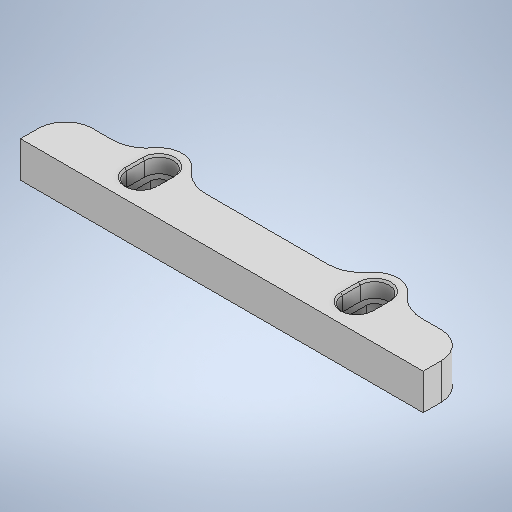
# Autodesk Inventor part: Montagemodul
Saved by Autodesk Inventor 2025.2 (Build 292293000, 293)
## iProperties
Created: 2025-11-06
Part Number: Montagemodul
Material: Generisch
Document SubType Name: Modeling
Designer: leowa
Density: 1 g/cm^3
Appearance: Vorgabe
Author: leowa
Autodesk Inventor part; units mm, degrees
ref_plane "YZ Plane" through (0, 0, 0) normal (1, 0, 0) x (0, 1, 0)
ref_plane "XZ Plane" through (0, 0, 0) normal (0, 1, 0) x (-1, 0, 0)
ref_plane "XY Plane" through (0, 0, 0) normal (0, 0, 1) x (1, 0, 0)
sketch "Skizze1" plane through (0, 0, 0) normal (0, 1, 0) x (-1, 0, 0)
  line L0 (-56, 7.5) -> (56, 7.5)
  line L1 (56, 7.5) -> (56, -7.5)
  line L2 (56, -7.5) -> (-56, -7.5)
  line L3 (-56, -7.5) -> (-56, 7.5)
  line L4 (-56, 7.5) -> (56, -7.5) construction
  line L5 (56, 7.5) -> (-56, -7.5) construction
  point P0 (0, 0)
  dimension "d0" = 15
  dimension "d1" = 112
  constraints: 12 end point, 2 midpoint, 2 parallel, 1 horizontal, 1 perpendicular
  measures "d0" distance of L0.end L1.end
  measures "d1" distance of L1.end L2.end
extrude "Extrusion1" add sketch "Skizze1" along normal blind 10
sketch "Skizze2" plane through (0, 10, 0) normal (0, 1, 0) x (1, 0, 0)
  line L0 (0, 10.5) -> (0, -10.5) projected
  line L1 (78.4, 0) -> (-78.4, 0) projected
  point P0 (0, 0)
  point P1 (-30, 0)
  point P2 (30, 0)
  dimension "d4" = 60
  constraints: 2 point on line, 1 symmetric about line
  measures "d4" distance of point (30, 0) point (-30, 0)
hole "Bohrung1" at (-30, 10, 0) at (30, 10, 0) direction (0, -1, 0) diameter 4.5 end through all counterbore diameter 8 counterbore depth 4.5 clearance for "Inbusschraube DIN EN ISO 4762" size "M4" standard "DIN"
chamfer "Fasen1" distance 0.5 angle 45 2 edges at (-30, 10, -4) (30, 10, -4)
ref_plane "Arbeitsebene1" through (30, -103.4416, 0) normal (0, 0, 1) x (0, 1, 0)
split body "Trennen1" result two bodies by plane through (30, -103.4416, 0) normal (0, 0, 1) first body at (-18.6667, 3.3333, 7)
move or copy body "Verschieben1" bodies to move or copy 2 copy no translate (0, 0, 5)
sketch "Skizze4" plane through (30, -103.4416, 0) normal (0, 0, 1) x (0, 1, 0)
  line L0 (113.4416, 86) -> (113.4416, 64.5) projected
  line L1 (113.4416, 64.5) -> (112.9416, 64) projected
  line L2 (112.9416, 64) -> (108.9416, 64) projected
  line L3 (108.9416, 64) -> (108.9416, 62.25) projected
  line L4 (108.9416, 62.25) -> (103.4416, 62.25) projected
  line L5 (103.4416, 62.25) -> (103.4416, 86) projected
  line L6 (103.4416, 86) -> (113.4416, 86) projected
  line L7 (113.4416, 55.5) -> (113.4416, 4.5) projected
  line L8 (113.4416, 4.5) -> (112.9416, 4) projected
  line L9 (112.9416, 4) -> (108.9416, 4) projected
  line L10 (108.9416, 4) -> (108.9416, 2.25) projected
  line L11 (108.9416, 2.25) -> (103.4416, 2.25) projected
  line L12 (103.4416, 2.25) -> (103.4416, 57.75) projected
  line L13 (103.4416, 57.75) -> (108.9416, 57.75) projected
  line L14 (108.9416, 57.75) -> (108.9416, 56) projected
  line L15 (108.9416, 56) -> (112.9416, 56) projected
  line L16 (112.9416, 56) -> (113.4416, 55.5) projected
  line L17 (103.4416, -26) -> (103.4416, -2.25) projected
  line L18 (103.4416, -2.25) -> (108.9416, -2.25) projected
  line L19 (108.9416, -2.25) -> (108.9416, -4) projected
  line L20 (108.9416, -4) -> (112.9416, -4) projected
  line L21 (112.9416, -4) -> (113.4416, -4.5) projected
  line L22 (113.4416, -4.5) -> (113.4416, -26) projected
  line L23 (113.4416, -26) -> (103.4416, -26) projected
  point P0 (103.4416, 30)
extrude "Extrusion3" add sketch "Skizze4" along normal blind 5 bodies 3
combine bodies "Kombinieren2" operation type add bodies to combine 2 3
sketch "Skizze3" plane through (0, 10, 0) normal (0, 1, 0) x (1, 0, 0)
  circle A0 centre (30, 0) radius 6.5
  line L0 (0, 0) -> (23.5, 0)
  arc A1 (16.8756, 0) -> (24.8298, 3.9394) centre (16.8756, 10) ccw
  line L1 (30, -5) -> (30, 18.5494)
  line L2 (56.0888, 0) -> (36.5, 0)
  arc A2 (35.1702, 3.9394) -> (43.1244, 0) centre (43.1244, 10) ccw
  line L3 (0, 24.7593) -> (0, -18.7099) projected
  circle A3 centre (-30, 0) radius 6.5
  line L4 (0, 0) -> (-23.5, 0)
  arc A4 (-24.8298, 3.9394) -> (-16.8756, 0) centre (-16.8756, 10) ccw
  line L5 (-30, -5) -> (-30, 18.5494)
  line L6 (-56.0888, 0) -> (-36.5, 0)
  arc A5 (-43.1244, 0) -> (-35.1702, 3.9394) centre (-43.1244, 10) ccw
  arc A6 (34.5, 0) -> (25.5, 0) centre (30, 0) ccw projected
  line L7 (56, -12.5) -> (56, 7.5) projected
  line L8 (56, 7.5) -> (-56, 7.5) projected
  arc A7 (-25.5, 0) -> (-34.5, 0) centre (-30, 0) ccw projected
  line L9 (-56, 7.5) -> (-56, -12.5) projected
  line L10 (34.5, 0) -> (34.5, -5) projected
  line L11 (-34.5, 0) -> (-34.5, -5) projected
  line L12 (-25.5, 0) -> (-25.5, -5) projected
  line L13 (25.5, 0) -> (25.5, -5) projected
  line L14 (-56, -12.5) -> (56, -12.5) projected
  arc A8 (-34.5, -5) -> (-25.5, -5) centre (-30, -5) ccw projected
  arc A9 (25.5, -5) -> (34.5, -5) centre (30, -5) ccw projected
  point P0 (-35.1702, 3.9394)
  point P1 (35.1702, 3.9394)
  point P2 (56, 0)
  point P3 (-24.8992, 4.0289)
  point P4 (-34.087, 5.0544)
  point P5 (23.6503, -1.3895)
  point P6 (35.8871, -2.7553)
  point P7 (-34.5, -4.6904)
  point P8 (25.5, -1.596)
  point P9 (-25.5, -4.6904)
  point P10 (34.5, -2.6004)
  point P11 (-56, 0)
  dimension "d16" = 10
  dimension "d24" = 2
  constraints: 15 symmetric about line, 14 point on circle, 12 end point, 6 centre point, 3 point on line, 2 horizontal, 2 tangent, 1 collinear, 1 concentric, 1 vertical, 4 other
  measures "d16" radius of A1
  measures "d24" radial gap between concentric circles of A6 A0
extrude "Extrusion2" cut sketch "Skizze3" against normal through all contours A0 L1 L8 L7 L2 A2 | A0 A1 L0 L3 L8 L1 | L3 L4 A4 A3 L5 L8 | L5 A3 A5 L6 L9 L8 bodies 2
fillet "Rundung1" radius 7.5 2 edges at (-56, 5, 0) (56, 5, 0)
equation "\"d0\" = Montage_Modulbreite"
equation "\"d2\" = Montage_Modulstärke"
equation "\"d4\" = Montage_Bohrungsabstand"
equation "\"d22\" = Montage_Langloch"
equation "\"d25\" = 0.5 * Montage_Modulbreite"
equation "\"d21\" = Montage_Langloch"
equation "\"Wandstärke\" = 3"
equation "\"Basisstärke\" = 3"
equation "\"Modulüberlappung\" = 2"
equation "\"Platinendicke\" = 1.8"
equation "\"Deckelstärke\" = 3"
equation "\"Seitenwand_Höhe\" = 39"
equation "\"Platinenposition\" = 5"
equation "\"Deckel_Klippbreite\" = 5"
equation "\"Deckel_Klipperposition\" = 4"
equation "\"Deckel_Klipperstärke\" = 1.5"
equation "\"Deckel_Klipptiefe\" = 1.5"
equation "\"Modul_Klipplänge\" = 8"
equation "\"Modul_Klipperposition\" = 7"
equation "\"Modul_Klipperstärke\" = 1.5"
equation "\"Modul_Klipptiefe\" = 1.5"
equation "\"Lüftungsraster\" = 2"
equation "\"Dings\" = 2"
equation "\"Generische_Modulbreite\" = 15"
equation "\"Relais_Modulbreite\" = 28"
equation "\"Modul_Grundflächenlänge\" = 102"
equation "\"Steckverbinder_Absatztiefe\" = 4"
equation "\"Steckverbinder_Absatzbreite\" = 2"
equation "\"Steckverbinder_Lochtiefe\" = 9"
equation "\"Steckverbinder_Fasenbreite\" = 1"
equation "\"Hauptmodul_Klipperabstand\" = 15"
equation "\"Stecktoleranz\" = 0.5"
equation "\"Deckel_Einrastführungslänge\" = 4"
equation "\"Deckel_Verstärkung\" = 2"
equation "\"Hauptmodul_Stufenposition\" = 53"
equation "\"Generische_Platinenhöhe\" = 38"
equation "\"Hauptmodul_Platinenhöhe_kurz\" = 48"
equation "\"Hauptmodul_Platinenhöhe_lang\" = 61"
equation "\"Hauptmodulbreite\" = 28"
equation "\"Montage_Bohrung\" = 4.5"
equation "\"Montage_Modulbreite\" = 15"
equation "\"Montage_Modulstärke\" = 10"
equation "\"Montage_Bohrungsabstand\" = 60"
equation "\"Montage_Langloch\" = 5"
equation "\"Deckklipper_Kantenverrundung\" = 1"
equation "\"Deckelklipper_Radius\" = 4"
equation "\"Modul_Klipperradius\" = 2"
equation "\"Modul_Klipper_Kantenverrundung\" = 1"
equation "\"Montage_Schwalbenschwanz_Länge\" = 3"
equation "\"Montage_Schwalbenschwanz_Winkel\" = 30deg"
equation "\"Test_Schnittabstand\" = 5"
equation "\"Hauptmodul_Deckel_Einschubtiefe\" = 2"
